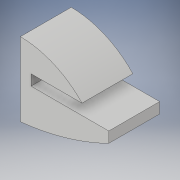
# Autodesk Inventor part: opticmount
Saved by Autodesk Inventor 2019.3 (Build 233278000, 278)
## iProperties
Created: 2019-04-14
Part Number: opticmount
Material: Generic
Document SubType Name: Modeling
Designer: peter
Density: 1 g/cm^3
Appearance: Default
Author: peter
Autodesk Inventor part; units mm, degrees
ref_plane "YZ Plane" through (0, 0, 0) normal (1, 0, 0) x (0, 1, 0)
ref_plane "XZ Plane" through (0, 0, 0) normal (0, 1, 0) x (-1, 0, 0)
ref_plane "XY Plane" through (0, 0, 0) normal (0, 0, 1) x (1, 0, 0)
sketch "Sketch1" plane through (0, 0, 0) normal (0, 0, 1) x (1, 0, 0)
  line L0 (0, -0.003) -> (0, -27.5)
  line L1 (0, -0.003) -> (0, -10) construction
  line L2 (0, -10) -> (4, -10) construction
  line L3 (4, -10) -> (4, -14)
  line L4 (4, -10) -> (23, -10)
  line L5 (4, -10) -> (23, -10) construction
  line L6 (4, -14) -> (33, -14)
  line L7 (33, -14) -> (33, -18)
  arc A0 (0, -27.5) -> (33, -18) centre (-9.9113, 68.9946) ccw
  line L8 (23, -10) -> (23, -10)
  line L9 (0, 0) -> (0, 0)
  arc A1 (23, -10) -> (0.0023, -0.003) centre (-0.1784, -31.8697) ccw
  line L10 (0, -0.003) -> (0, -10)
  line L11 (0, -10) -> (23, -10)
  line L12 (0.0023, -0.003) -> (0, -0.003)
  dimension "d0" = 27.5
  dimension "d1" = 10
  dimension "d2" = 4
  dimension "d3" = 4
  dimension "d4" = 19
  dimension "d5" = 0
  dimension "d6" = 29
  dimension "d7" = 4
  constraints: 26 end point, 4 horizontal, 4 perpendicular, 4 point on circle, 2 centre point, 2 collinear, 2 point on line, 1 vertical
  measures "d0" distance of L9.start L0.end
  measures "d1" distance of L9.start L1.end
  measures "d2" distance of L1.end L2.end
  measures "d3" distance of L2.end L3.end
  measures "d4" distance of L2.end L4.end
  measures "d5" distance between parallel lines of L4 L5
  measures "d6" distance of L3.end L6.end
  measures "d7" distance of L6.end L7.end
extrude "Extrusion1" add sketch "Sketch1" along normal blind 19
body "Solid1"
